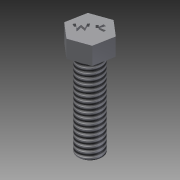
# Autodesk Inventor part: 1in bolt
Saved by Autodesk Inventor 2011 SP1 (Build 150282100, 282)
## iProperties
Created: 2013-01-18
Part Number: 1in bolt
Document SubType Name: Modeling
Designer: wes
Density: 1 g/cm^3
Author: wes
Autodesk Inventor part; units mm, degrees
ref_plane "YZ Plane" through (0, 0, 0) normal (1, 0, 0) x (0, 1, 0)
ref_plane "XZ Plane" through (0, 0, 0) normal (0, 1, 0) x (-1, 0, 0)
ref_plane "XY Plane" through (0, 0, 0) normal (0, 0, 1) x (1, 0, 0)
sketch "Sketch1" plane through (0, 0, 0) normal (0, 0, 1) x (1, 0, 0)
  line L0 (-2.7545, 0) -> (0.6745, 0)
  line L1 (0.6745, 0) -> (0.6745, 25.4)
  line L2 (0.6745, 25.4) -> (-2.7545, 25.4)
  line L3 (-2.7545, 25.4) -> (-2.7545, 0)
  point P0 (0, 0)
  dimension "d0" = 3.429
  dimension "d1" = 25.4
  constraints: 8 end point, 2 parallel, 1 horizontal, 1 perpendicular
  measures "d0" distance of L0.start L0.end
  measures "d1" distance of L0.end L1.end
revolve "Revolution1" add sketch "Sketch1" angle 360 about axis through (-2.7545, 25.4, 0) along (0, -1, 0)
sketch "Sketch2" plane through (-2.7545, 25.4, 0) normal (0, 1, 0) x (1, 0, 0)
  circle A0 centre (0, 0) radius 3.429 projected
  line L0 (-1.0753, -5.7665) -> (-5.5316, -1.952)
  line L1 (-5.5316, -1.952) -> (-4.4562, 3.8145)
  line L2 (-4.4562, 3.8145) -> (1.0753, 5.7665)
  line L3 (1.0753, 5.7665) -> (5.5316, 1.952)
  line L4 (5.5316, 1.952) -> (4.4562, -3.8145)
  line L5 (4.4562, -3.8145) -> (-1.0753, -5.7665)
  point P0 (2.7545, 0)
  dimension "d3" = 5.08
  constraints: 12 end point, 1 coincident, 13 other
  measures "d3" distance from line of A0.centre L1
extrude "Extrusion1" add sketch "Sketch2" along normal blind 5.08 contours A0 | L0 L1 L2 L3 L4 L5
thread "Thread1" size "5/16-18 UNC" class "2A" standard "ANSI Unified Screw Threads" full length
sketch "Sketch3" plane through (-2.7545, 30.48, 0) normal (0, 1, 0) x (1, 0, 0)
  line L0 (5.5316, 1.952) -> (4.4562, -3.8145) projected
  line L1 (1.0753, 5.7665) -> (5.5316, 1.952) projected
  line L2 (-4.4562, 3.8145) -> (1.0753, 5.7665) projected
  line L3 (-3.9194, -1.1734) -> (-1.366, -2.4875)
  line L4 (-1.366, -2.4875) -> (-1.2813, -2.3228)
  line L5 (-1.2813, -2.3228) -> (-1.7974, -0.8601)
  line L6 (-1.7974, -0.8601) -> (-0.2306, -1.1523)
  line L7 (-0.2306, -1.1523) -> (0.0392, -0.6281)
  line L8 (0.0392, -0.6281) -> (-1.4654, 1.4765)
  line L9 (-1.4654, 1.4765) -> (-1.8516, 1.0253)
  line L10 (-1.8516, 1.0253) -> (-1.0682, -0.4113)
  line L11 (-1.0682, -0.4113) -> (-2.4324, -0.1569)
  line L12 (-2.4324, -0.1569) -> (-2.1392, -1.7523)
  line L13 (-2.1392, -1.7523) -> (-3.4526, -0.6281)
  line L14 (-3.4526, -0.6281) -> (-3.9194, -1.1734)
  line L15 (-0.2889, 1.952) -> (1.6905, 0)
  line L16 (1.6905, 0) -> (1.9932, 0.307)
  line L17 (1.9932, 0.307) -> (1.0361, 1.2509)
  line L18 (1.0361, 1.2509) -> (2.6233, 1.3796)
  line L19 (2.6233, 1.3796) -> (2.569, 2.0493)
  line L20 (2.569, 2.0493) -> (1.0361, 1.7676)
  line L21 (1.0361, 1.7676) -> (1.5146, 3.1041)
  line L22 (1.5146, 3.1041) -> (0.7008, 3.2559)
  line L23 (0.7008, 3.2559) -> (0.6427, 1.9085)
  line L24 (0.6427, 1.9085) -> (0.1487, 2.3957)
  line L25 (0.1487, 2.3957) -> (-0.2889, 1.952)
  point P0 (2.7545, 0)
  constraints: 46 end point, 9 perpendicular, 6 parallel
extrude "Extrusion2" cut sketch "Sketch3" against normal blind 0.762
body "Solid1"
